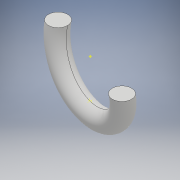
# Autodesk Inventor part: spring_part
Saved by Autodesk Inventor 2017.2 (Build 212233000, 233)
## iProperties
Created: 2017-08-28
Part Number: spring_part
Material: Generic
Document SubType Name: Modeling
Designer: Nic
Density: 1 g/cm^3
Appearance: Default
Author: Nic
Autodesk Inventor part; units mm, degrees
ref_plane "YZ Plane" through (0, 0, 0) normal (1, 0, 0) x (0, 1, 0)
ref_plane "XZ Plane" through (0, 0, 0) normal (0, 1, 0) x (-1, 0, 0)
sketch "Sketch1" plane through (0, 0, 0) normal (0, 0, 1) x (1, 0, 0)
  line L0 (0, 12.3589) -> (0, 0)
  line L1 (-3, 0) -> (3, 0)
  circle A0 centre (-3, 0.6) radius 0.6
  dimension "d1" = 1.2
  dimension "d10" = 6
  constraints: 4 end point, 1 centre point, 1 horizontal, 1 midpoint, 1 tangent, 1 vertical, 1 vertical alignment
  measures "d1" diameter of A0
  measures "d10" distance of L1.start L1.end
coil "Coil1" sketch "Sketch1" operation add axis through (0, 12.3589, 0) along (0, -1, 0) pitch 4 turns 0.5 hand right
sketch "Sketch2" plane through (-3, 0.6, 0) normal (0, 0, 1) x (1, 0, 0)
  circle A0 centre (0, 0) radius 0.6 projected
  circle A1 centre (6, -2) radius 0.6 projected
  line L0 (0, 0) -> (6, -2)
  line L1 (6, -2) -> (-0.1349, -0.5846)
  line L2 (3, -1) -> (2.9326, -1.2923)
  point P0 (3, -0.6)
  point P1 (0.6, 0)
  point P2 (6.9451, -2.5)
  point P3 (5.4, -2)
  constraints: 6 end point, 2 midpoint, 1 horizontal alignment, 1 point on circle, 1 tangent, 1 other
sketch3d "3D Sketch1"
ref_plane "Work Plane1" through (-3, 0.6, 0) normal (0.3162, 0.9487, 0) x (0.9487, -0.3162, 0)
body "Solid1"
